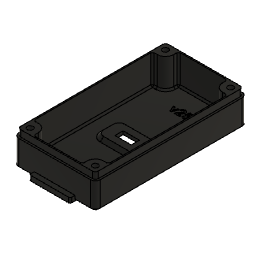
Back_Lid_M1 (Autodesk Fusion 360 design; units mm, degrees)
Autodesk Fusion 360 part; units mm, degrees
note: some values were not read from the file. Set by a fixed rule: which face or edge a step refers to.
sketch "Skizze1" plane through (0, 0, 0) normal (0, 0, 1) x (1, 0, 0)
  line L0 (-22, -46.5) -> (22, -46.5)
  line L1 (25, -43.5) -> (25, 43.5)
  line L2 (22, 46.5) -> (-22, 46.5)
  line L3 (-25, 43.5) -> (-25, -43.5)
  line L4 (-25, -46.5) -> (25, 46.5) construction
  line L5 (25, -46.5) -> (-25, 46.5) construction
  arc A0 (25, 43.5) -> (22, 46.5) centre (22, 43.5) ccw
  arc A1 (-22, 46.5) -> (-25, 43.5) centre (-22, 43.5) ccw
  arc A2 (-25, -43.5) -> (-22, -46.5) centre (-22, -43.5) ccw
  arc A3 (22, -46.5) -> (25, -43.5) centre (22, -43.5) ccw
  dimension "d116" = 50
  dimension "d117" = 93
  dimension "d118" = 3
  constraint horizontal L0
  constraint perpendicular L0 L1
  constraint parallel L0 L2
  constraint parallel L1 L3
  constraint coincident L4 origin
  constraint coincident L5 origin
  constraint coincident L4.end L1
  constraint coincident L4.end L2
  constraint tangent L1 A0
  constraint tangent L2 A0
  constraint coincident L5.end L2
  constraint coincident L5.end L3
  constraint tangent L2 A1
  constraint tangent L3 A1
  constraint equal A0 A1
  constraint coincident L4.start L3
  constraint coincident L4.start L0
  constraint tangent L3 A2
  constraint tangent L0 A2
  constraint equal A0 A2
  constraint coincident L5.start L0
  constraint coincident L5.start L1
  constraint tangent L0 A3
  constraint tangent L1 A3
  constraint equal A0 A3
  measures "d116" distance of L4.end L5.end
  measures "d117" distance of L5.start L4.end
  measures "d118" radius of A0
extrude "Extrusion1" add sketch "Skizze1" along normal blind 20 makes body 1
shell "Schale1" thickness 2 removed faces 1 at (-8.3333, 14.5, 20) on bodies 1
sketch "Skizze6" plane through (0, 0, 20) normal (0, 0, 1) x (-1, 0, 0)
  line L0 (-22, 44.5) -> (22, 44.5)
  arc A0 (23, 43.5) -> (22, 44.5) centre (22, 43.5) ccw
  line L1 (23, 43.5) -> (23, -43.5)
  arc A1 (22, -44.5) -> (23, -43.5) centre (22, -43.5) ccw
  line L2 (22, -44.5) -> (-22, -44.5)
  arc A2 (-23, -43.5) -> (-22, -44.5) centre (-22, -43.5) ccw
  line L3 (-23, -43.5) -> (-23, 43.5)
  arc A3 (-22, 44.5) -> (-23, 43.5) centre (-22, 43.5) ccw
  arc A4 (-22, 46.5) -> (-25, 43.5) centre (-22, 43.5) ccw
  line L4 (-25, 43.5) -> (-25, -43.5)
  arc A5 (-25, -43.5) -> (-22, -46.5) centre (-22, -43.5) ccw
  line L5 (-22, -46.5) -> (22, -46.5)
  arc A6 (22, -46.5) -> (25, -43.5) centre (22, -43.5) ccw
  line L6 (25, -43.5) -> (25, 43.5)
  arc A7 (25, 43.5) -> (22, 46.5) centre (22, 43.5) ccw
  line L7 (22, 46.5) -> (-22, 46.5)
  line L8 (-23.8, 43.5) -> (-23.8, -43.5)
  arc A8 (-23.8, -43.5) -> (-22, -45.3) centre (-22, -43.5) ccw
  line L9 (-22, -45.3) -> (22, -45.3)
  arc A9 (22, -45.3) -> (23.8, -43.5) centre (22, -43.5) ccw
  line L10 (23.8, -43.5) -> (23.8, 43.5)
  arc A10 (23.8, 43.5) -> (22, 45.3) centre (22, 43.5) ccw
  line L11 (22, 45.3) -> (-22, 45.3)
  arc A11 (-22, 45.3) -> (-23.8, 43.5) centre (-22, 43.5) ccw
  dimension "d305" = -1.2
extrude "Extrusion5" cut sketch "Skizze6" against normal blind 4 contours A4 L4 A5 L5 A6 L6 A7 L7 bodies 1
sketch "Skizze8" plane through (0, 0, 2) normal (0, 0, 1) x (-1, 0, 0)
  arc A0 (-22, 44.5) -> (-23, 43.5) centre (-22, 43.5) ccw
  line L0 (-23, 43.5) -> (-23, -43.5)
  arc A1 (-23, -43.5) -> (-22, -44.5) centre (-22, -43.5) ccw
  line L1 (-22, -44.5) -> (22, -44.5)
  arc A2 (22, -44.5) -> (23, -43.5) centre (22, -43.5) ccw
  line L2 (23, -43.5) -> (23, 43.5)
  arc A3 (23, 43.5) -> (22, 44.5) centre (22, 43.5) ccw
  line L3 (22, 44.5) -> (-22, 44.5)
  line L4 (20, -36.5) -> (23, -36.5)
  line L5 (15, -41.5) -> (15, -44.5)
  arc A4 (20, -36.5) -> (15, -41.5) centre (20, -41.5) ccw
  line L6 (-15, -41.5) -> (-15, -44.5)
  line L7 (-20, -36.5) -> (-23, -36.5)
  arc A5 (-15, -41.5) -> (-20, -36.5) centre (-20, -41.5) ccw
  line L8 (-15, 41.5) -> (-15, 44.5)
  line L9 (-20, 36.5) -> (-23, 36.5)
  line L10 (20, 36.5) -> (23, 36.5)
  line L11 (15, 41.5) -> (15, 44.5)
  arc A6 (-20, 36.5) -> (-15, 41.5) centre (-20, 41.5) ccw
  arc A7 (15, 41.5) -> (20, 36.5) centre (20, 41.5) ccw
  dimension "d314" = 40
  dimension "d315" = 5
  constraint coincident L2 L4.end
  constraint perpendicular L2 L4
  constraint coincident L1 L5.end
  constraint perpendicular L1 L5
  constraint tangent L5 A4
  constraint tangent L4 A4
  constraint coincident L1 L6.end
  constraint perpendicular L1 L6
  constraint coincident L0 L7.end
  constraint perpendicular L0 L7
  constraint tangent L6 A5
  constraint tangent L7 A5
  constraint horizontal A4.centre A5.centre
  constraint horizontal L4.start L7.start
  constraint equal L4 L5
  constraint equal L6 L7
  constraint coincident L3 L8.end
  constraint perpendicular L3 L8
  constraint coincident L0 L9.end
  constraint perpendicular L0 L9
  constraint coincident L2 L10.end
  constraint perpendicular L2 L10
  constraint coincident L3 L11.end
  constraint perpendicular L3 L11
  constraint tangent L10 A7
  constraint tangent L11 A7
  constraint tangent L8 A6
  constraint tangent L9 A6
  constraint equal L10 L11
  constraint equal L8 L9
  constraint equal A4 A7
  constraint equal A4 A6
  constraint vertical A4.centre A7.centre
  constraint vertical A5.centre A6.centre
  measures "d314" distance of A4.centre A5.centre
  measures "d315" radius of A4
extrude "Extrusion6" add sketch "Skizze8" along normal up to surface (18 mm away) contours A0 L0 L3 L8 L9 A6 | L2 A3 L3 L10 L11 A7 | L0 A1 L1 L6 L7 A5 | L1 A2 L2 L4 L5 A4 bodies 1
sketch "Skizze7" plane through (0, 0, 0) normal (0, 0, -1) x (1, 0, 0)
  arc A0 (25, 43.5) -> (22, 46.5) centre (22, 43.5) ccw
  line L0 (22, 46.5) -> (-22, 46.5)
  arc A1 (-22, 46.5) -> (-25, 43.5) centre (-22, 43.5) ccw
  line L1 (-25, 43.5) -> (-25, -43.5)
  arc A2 (-25, -43.5) -> (-22, -46.5) centre (-22, -43.5) ccw
  line L2 (-22, -46.5) -> (22, -46.5)
  arc A3 (22, -46.5) -> (25, -43.5) centre (22, -43.5) ccw
  line L3 (25, -43.5) -> (25, 43.5)
  point P0 (20, -41.5)
  point P1 (-20, -41.5)
  point P2 (20, 41.5)
  point P3 (-20, 41.5)
  dimension "d308" = 83
  dimension "d309" = 41.5
  dimension "d310" = 40
  dimension "d311" = 20
  constraint horizontal P0 P1
  constraint horizontal P2 P3
  constraint vertical P0 P2
  constraint vertical P1 P3
  measures "d308" distance of P0 P2
  measures "d309" vertical distance of origin P0
  measures "d310" distance of P0 P1
  measures "d311" horizontal distance of origin P0
hole "Bohrung2" at (20, 41.5, 0) at (-20, 41.5, 0) at (-20, -41.5, 0) at (20, -41.5, 0) direction (0, 0, 1) diameter 3.5 end up to surface (20 mm away) countersink diameter 6 countersink angle 90 bodies 1
ref_plane "Arbeitsebene1" through (0, 0, 0) normal (0, 0, -1) x (-1, 0, 0)
sketch "Skizze9" plane through (0, 0, 0) normal (0, 0, -1) x (-1, 0, 0)
  line L0 (-22, -46.5) -> (22, -46.5)
  line L1 (12.5, -46.5) -> (-12.5, -46.5)
  line L2 (-12.5, -46.5) -> (-12.5, -48.5)
  line L3 (-11.5, -49.5) -> (11.5, -49.5)
  line L4 (12.5, -48.5) -> (12.5, -46.5)
  arc A0 (11.5, -49.5) -> (12.5, -48.5) centre (11.5, -48.5) ccw
  arc A1 (-12.5, -48.5) -> (-11.5, -49.5) centre (-11.5, -48.5) ccw
  line L5 (22, -46.5) -> (-22, -46.5)
  line L6 (-22, 46.5) -> (22, 46.5)
  point P0 (-12.5, -49.5)
  point P1 (12.5, -49.5)
  dimension "d379" = 25
  dimension "d380" = 12.5
  dimension "d381" = 3
  dimension "d382" = 1
  constraint horizontal L1
  constraint vertical L2
  constraint horizontal L3
  constraint vertical L4
  constraint coincident P1 L4
  constraint coincident P1 L3
  constraint tangent L4 A0
  constraint tangent L3 A0
  constraint coincident P0 L3
  constraint coincident P0 L2
  constraint tangent L3 A1
  constraint tangent L2 A1
  constraint equal A0 A1
  constraint horizontal L0.end L1.start
  measures "d379" distance of P0 P1
  measures "d380" distance of origin L4
  measures "d381" distance of L1.end P0
  measures "d382" radius of A0
extrude "Extrusion7" add sketch "Skizze9" against normal blind 3 bodies 1
sketch "Skizze10" plane through (0, 0, 2) normal (0, 0, 1) x (-1, 0, 0)
  line L0 (5.5, -28.5) -> (-5.5, -28.5) construction
  line L1 (-5.5, -28.5) -> (-5.5, -33.5) construction
  line L2 (-5.5, -33.5) -> (5.5, -33.5) construction
  line L3 (5.5, -33.5) -> (5.5, -28.5) construction
  line L4 (23, 36.5) -> (20, 36.5)
  arc A0 (15, 41.5) -> (20, 36.5) centre (20, 41.5) ccw
  line L5 (15, 41.5) -> (15, 44.5)
  line L6 (15, 44.5) -> (-15, 44.5)
  line L7 (-15, 44.5) -> (-15, 41.5)
  arc A1 (-20, 36.5) -> (-15, 41.5) centre (-20, 41.5) ccw
  line L8 (-20, 36.5) -> (-23, 36.5)
  line L9 (-23, 36.5) -> (-23, -36.5)
  line L10 (-23, -36.5) -> (-20, -36.5)
  arc A2 (-15, -41.5) -> (-20, -36.5) centre (-20, -41.5) ccw
  line L11 (-15, -41.5) -> (-15, -44.5)
  line L12 (-15, -44.5) -> (15, -44.5)
  line L13 (15, -44.5) -> (15, -41.5)
  arc A3 (20, -36.5) -> (15, -41.5) centre (20, -41.5) ccw
  line L14 (20, -36.5) -> (23, -36.5)
  line L15 (23, -36.5) -> (23, 36.5)
  dimension "d393" = 5
  dimension "d394" = 5
  dimension "d396" = 11
  text T0 "v25" font "Arial" height 5 bold align centre middle in box 11 x 5 at (5.5, -28.5) x (-1, 0) y (0, -1) spacing 1 kerned
  constraint vertical origin
extrude "Extrusion8" cut sketch "Skizze10" against normal blind 0.3 text T0 bodies 1
sketch "Skizze11" plane through (0, 0, 0) normal (0, 0, -1) x (1, 0, 0)
  line L0 (-12.5, 48.5) -> (-12.5, 46.5)
  line L1 (12.5, 46.5) -> (12.5, 48.5)
  arc A0 (12.5, 48.5) -> (11.5, 49.5) centre (11.5, 48.5) ccw
  line L2 (11.5, 49.5) -> (-11.5, 49.5)
  arc A1 (-11.5, 49.5) -> (-12.5, 48.5) centre (-11.5, 48.5) ccw
  circle A2 centre (20, 41.5) radius 3
  circle A3 centre (-20, -41.5) radius 3
  circle A4 centre (20, -41.5) radius 3
  circle A5 centre (-20, 41.5) radius 3
  line L3 (-9, 6) -> (7, 6)
  line L4 (9, 4) -> (9, -2)
  line L5 (7, -4) -> (-9, -4)
  line L6 (-11, -2) -> (-11, 4)
  line L7 (-11, 6) -> (9, -4) construction
  line L8 (9, 6) -> (-11, -4) construction
  line L9 (-6, 3.5) -> (4, 3.5)
  line L10 (4, 3.5) -> (4, -1.5)
  line L11 (4, -1.5) -> (-6, -1.5)
  line L12 (-6, -1.5) -> (-6, 3.5)
  line L13 (-6, 3.5) -> (4, -1.5) construction
  line L14 (4, 3.5) -> (-6, -1.5) construction
  line L15 (-9, 7.5) -> (7, 7.5)
  line L16 (10.5, 4) -> (10.5, -2)
  line L17 (7, -5.5) -> (-9, -5.5)
  line L18 (-12.5, -2) -> (-12.5, 4)
  line L19 (-12.5, 7.5) -> (10.5, -5.5) construction
  line L20 (10.5, 7.5) -> (-12.5, -5.5) construction
  arc A6 (-9, 6) -> (-11, 4) centre (-9, 4) ccw
  arc A7 (9, 4) -> (7, 6) centre (7, 4) ccw
  arc A8 (7, -4) -> (9, -2) centre (7, -2) ccw
  arc A9 (-11, -2) -> (-9, -4) centre (-9, -2) ccw
  arc A10 (-9, 7.5) -> (-12.5, 4) centre (-9, 4) ccw
  arc A11 (10.5, 4) -> (7, 7.5) centre (7, 4) ccw
  arc A12 (7, -5.5) -> (10.5, -2) centre (7, -2) ccw
  arc A13 (-12.5, -2) -> (-9, -5.5) centre (-9, -2) ccw
  arc A14 (25, 43.5) -> (22, 46.5) centre (22, 43.5) ccw
  line L21 (22, 46.5) -> (12.5, 46.5)
  line L22 (-12.5, 46.5) -> (-22, 46.5)
  arc A15 (-22, 46.5) -> (-25, 43.5) centre (-22, 43.5) ccw
  line L23 (-25, 43.5) -> (-25, -43.5)
  arc A16 (-25, -43.5) -> (-22, -46.5) centre (-22, -43.5) ccw
  line L24 (-22, -46.5) -> (22, -46.5)
  arc A17 (22, -46.5) -> (25, -43.5) centre (22, -43.5) ccw
  line L25 (25, -43.5) -> (25, 43.5)
  line L26 (0.8, 1.82) -> (0.8, 0.18)
  line L27 (0.8, 0.18) -> (-2.8, 0.18)
  line L28 (-2.8, 0.18) -> (-2.8, 1.82)
  line L29 (-2.8, 1.82) -> (0.8, 1.82)
  line L30 (3.25, 2.75) -> (-5.25, 2.75)
  line L31 (-5.25, 2.75) -> (-5.25, -0.75)
  line L32 (-5.25, -0.75) -> (3.25, -0.75)
  line L33 (3.25, -0.75) -> (3.25, 2.75)
  line L34 (3.25, -0.75) -> (-5.25, 2.75)
  point P0 (-1, 1)
  point P1 (-1, 1)
  point P2 (-1, 1)
  point P3 (-1, 1)
  point P4 (-1, 1)
  point P5 (-1, 1)
  dimension "d451" = 10
  dimension "d452" = 20
  dimension "d455" = 10
  dimension "d456" = 5
  dimension "d457" = 1.5
  dimension "d458" = 1.5
  dimension "d462" = 2
  dimension "d463" = 3.5
  constraint horizontal L3
  constraint perpendicular L3 L4
  constraint parallel L3 L5
  constraint parallel L4 L6
  constraint coincident L7 P5
  constraint coincident L8 P5
  constraint coincident P5 P4
  constraint horizontal L9
  constraint perpendicular L9 L10
  constraint parallel L9 L11
  constraint parallel L10 L12
  constraint coincident L13 P5
  constraint coincident L14 P5
  constraint horizontal L15
  constraint perpendicular L15 L16
  constraint parallel L15 L17
  constraint parallel L16 L18
  constraint coincident L19 P5
  constraint coincident L20 P5
  constraint coincident L7.start L6
  constraint coincident L7.start L3
  constraint tangent L6 A6
  constraint tangent L3 A6
  constraint coincident L8.start L3
  constraint coincident L8.start L4
  constraint tangent L3 A7
  constraint tangent L4 A7
  constraint equal A6 A7
  constraint coincident L7.end L4
  constraint coincident L7.end L5
  constraint tangent L4 A8
  constraint tangent L5 A8
  constraint equal A6 A8
  constraint coincident L8.end L5
  constraint coincident L8.end L6
  constraint tangent L5 A9
  constraint tangent L6 A9
  constraint equal A6 A9
  constraint coincident L19.start L18
  constraint coincident L19.start L15
  constraint tangent L18 A10
  constraint tangent L15 A10
  constraint coincident L20.start L15
  constraint coincident L20.start L16
  constraint tangent L15 A11
  constraint tangent L16 A11
  constraint equal A10 A11
  constraint coincident L19.end L16
  constraint coincident L19.end L17
  constraint tangent L16 A12
  constraint tangent L17 A12
  constraint equal A10 A12
  constraint coincident L20.end L17
  constraint coincident L20.end L18
  constraint tangent L17 A13
  constraint tangent L18 A13
  constraint equal A10 A13
  constraint coincident L32.end L33.start
  constraint coincident L30.end L31.start
  constraint midpoint L34 P5
  measures "d451" distance of L7.start L8.end
  measures "d452" distance of L7.end L8.end
  measures "d455" distance of L10.end L11.end
  measures "d456" distance of L9.end L10.end
  measures "d457" distance of L4 L16
  measures "d458" distance of L3 L15
  measures "d462" radius of A6
  measures "d463" radius of A10
extrude "Extrusion9" add sketch "Skizze11" against normal blind 4 contours L3 L4 L5 L6 A6 A7 A8 A9 | L15 L16 L17 L18 A10 A11 A12 A13 bodies 1
extrude "Extrusion10" cut sketch "Skizze11" against normal up to surface (2 mm away) contours L3 L4 L5 L6 A6 A7 A8 A9 | L9 L10 L11 L12 | L26 L28 L29 L30 L33 L34 | L26 L28 L29 L34 | L26 L27 L28 L31 L32 L34 | L26 L27 L28 L34 bodies 1
chamfer "Fase1" distance 1 angle 45 33 edges at (17.25, -46.5, 0) (24.1213, -45.6213, 0) (25, 0, 0) (24.1213, 45.6213, 0) (0, 46.5, 0) (-24.1213, 45.6213, 0) (-25, 0, 0) (-24.1213, -45.6213, 0) (-17.25, -46.5, 0) (16.4645, 37.9645, 2) (21.5, 36.5, 2) (15, 43, 2) (-16.4645, 37.9645, 2) (-15, 43, 2) (-21.5, 36.5, 2) (0, 44.5, 2) (-23, 0, 2) (-16.4645, -37.9645, 2) (-21.5, -36.5, 2) (-15, -43, 2) (0, -44.5, 2) (16.4645, -37.9645, 2) (15, -43, 2) (21.5, -36.5, 2) (23, 0, 2) (23, 36.5, 11) (15, 44.5, 11) (-15, 44.5, 11) (-23, 36.5, 11) (-23, -36.5, 11) (-15, -44.5, 11) (15, -44.5, 11) (23, -36.5, 11) on bodies 1
chamfer "Fase1" distance 2 angle 45 8 edges at (-1, -7.5, 2) (-11.4749, -6.4749, 2) (-12.5, -1, 2) (-11.4749, 4.4749, 2) (-1, 5.5, 2) (9.4749, 4.4749, 2) (10.5, -1, 2) (9.4749, -6.4749, 2) on bodies 1
chamfer "Fase1" distance 0.5 angle 45 8 edges at (-10.4142, 3.4142, 0) (-11, -1, 0) (-10.4142, -5.4142, 0) (-1, -6, 0) (8.4142, -5.4142, 0) (9, -1, 0) (8.4142, 3.4142, 0) (-1, 4, 0) on bodies 1
sketch "Skizze12" plane through (0, 0, 0) normal (0, 0, -1) x (1, 0, 0)
  circle A0 centre (-20, 41.5) radius 3
  circle A1 centre (20, -41.5) radius 3
  circle A2 centre (-20, -41.5) radius 3
  circle A3 centre (20, 41.5) radius 3
  line L0 (-12.5, 48.5) -> (-12.5, 45.5)
  line L1 (-12.5, 45.5) -> (-22, 45.5)
  arc A4 (-22, 45.5) -> (-24, 43.5) centre (-22, 43.5) ccw
  line L2 (-24, 43.5) -> (-24, -43.5)
  arc A5 (-24, -43.5) -> (-22, -45.5) centre (-22, -43.5) ccw
  line L3 (-22, -45.5) -> (22, -45.5)
  arc A6 (22, -45.5) -> (24, -43.5) centre (22, -43.5) ccw
  line L4 (24, -43.5) -> (24, 43.5)
  arc A7 (24, 43.5) -> (22, 45.5) centre (22, 43.5) ccw
  line L5 (22, 45.5) -> (12.5, 45.5)
  line L6 (12.5, 45.5) -> (12.5, 48.5)
  arc A8 (12.5, 48.5) -> (11.5, 49.5) centre (11.5, 48.5) ccw
  line L7 (11.5, 49.5) -> (-11.5, 49.5)
  arc A9 (-11.5, 49.5) -> (-12.5, 48.5) centre (-11.5, 48.5) ccw
  arc A10 (-11.5, -2) -> (-9, -4.5) centre (-9, -2) ccw
  line L8 (-11.5, -2) -> (-11.5, 4)
  arc A11 (-9, 6.5) -> (-11.5, 4) centre (-9, 4) ccw
  line L9 (-9, 6.5) -> (7, 6.5)
  arc A12 (9.5, 4) -> (7, 6.5) centre (7, 4) ccw
  line L10 (9.5, 4) -> (9.5, -2)
  arc A13 (7, -4.5) -> (9.5, -2) centre (7, -2) ccw
  line L11 (7, -4.5) -> (-9, -4.5)
  line L12 (15.5, 6.5) -> (10.5, 6.5) construction
  line L13 (10.5, 6.5) -> (10.5, -4.5) construction
  line L14 (10.5, -4.5) -> (15.5, -4.5) construction
  line L15 (15.5, -4.5) -> (15.5, 6.5) construction
  line L16 (-12.5, 6.5) -> (-17.5, 6.5) construction
  line L17 (-17.5, 6.5) -> (-17.5, -4.5) construction
  line L18 (-17.5, -4.5) -> (-12.5, -4.5) construction
  line L19 (-12.5, -4.5) -> (-12.5, 6.5) construction
  dimension "d511" = 7
  dimension "d512" = 1
  dimension "d513" = 5
  dimension "d514" = 7
  dimension "d515" = 1
  text T0 "1" font "Arial" height 7 bold align centre middle in box 5 x 11 at (15.5, 6.5) x (-1, 0) y (0, -1) spacing 1 kerned
  text T1 "0" font "Arial" height 7 bold align centre middle in box 5 x 11 at (-12.5, 6.5) x (-1, 0) y (0, -1) spacing 1 kerned
  constraint horizontal A13.start
  constraint horizontal L9.end
  constraint horizontal A10.end
  constraint horizontal A11.start
  constraint equal L14 L18
  measures "d512" distance of L10 L13
  measures "d515" distance of L8 L19
extrude "Extrusion11" cut sketch "Skizze12" against normal blind 0.5 text T0 T1 bodies 1
extrude "Extrusion1'" add 2 faces at (11.9097, -0.4716, 0.5) (-16.7905, -1.5447, 0.5) along direction (0, 0, -1) blind 0.5 separate body on bodies 1 makes body 2 at (11.9097, -0.4716, 0.5) makes body 3 at (-16.7905, -1.5447, 0.5) in component "Back_Lid_Text"
component "Back_Lid_Text" placed x (1, 0, 0) y (0, 1, 0) z (0, 0, 1) at (0, 0, 0)
equation "d309 = d308 / 2"
equation "d311 = d310 / 2"
equation "d380 = d379 / 2"
equation "d458 = d457"
equation "d463 = d462 + d457"
equation "d515 = d512"
named bodies: "Back_Lid"
